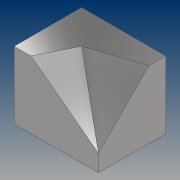
# Autodesk Inventor part: 24
Saved by Autodesk Inventor 2020.2 (Build 242310000, 310)
## iProperties
Created: 2020-09-17
Part Number: 24
Material: 鋼、碳鋼
Document SubType Name: Modeling
Designer: user
Density: 7.85 g/cm^3
Appearance: 半拋光
Mass: 561.275 g
Surface Area: 104.759 cm^2
Volume: 71.5 cm^3
Author: user
Autodesk Inventor part; units mm, degrees
ref_plane "YZ Plane" through (0, 0, 0) normal (1, 0, 0) x (0, 1, 0)
ref_plane "XZ Plane" through (0, 0, 0) normal (0, 1, 0) x (-1, 0, 0)
sketch "草圖1" plane through (0, 0, 0) normal (0, 1, 0) x (-1, 0, 0)
  line L0 (0, 0) -> (-50, 0)
  line L1 (-50, 0) -> (-50, -40)
  line L2 (-50, -40) -> (0, -40)
  line L3 (0, -40) -> (0, 0)
  dimension "d0" = 50
  dimension "d1" = 40
  constraints: 8 end point, 2 parallel, 1 horizontal, 1 perpendicular
  measures "d0" distance of L0.start L0.end
  measures "d1" distance of L2.end L0.start
extrude "擠出1" add sketch "草圖1" along normal blind 40
sketch "草圖2" plane through (0, 40, 0) normal (0, 1, 0) x (1, 0, 0)
  line L0 (0, 0) -> (0, 40) construction
  line L1 (0, 40) -> (50, 40) construction
  line L2 (50, 40) -> (50, 0) construction
  line L3 (50, 0) -> (0, 0) construction
  line L4 (0, 0) -> (50, 0) construction
  line L5 (10, 0) -> (20, 20)
  line L6 (20, 20) -> (50, 0)
  line L7 (10, 0) -> (50, 0)
  dimension "d4" = 20
  dimension "d5" = 40
  dimension "d6" = 10
  constraints: 6 end point, 1 collinear, 1 point on line
  measures "d4" distance from line of L5.end L3
  measures "d5" distance from line of L2 L5.start
  measures "d6" horizontal distance of L5.end L5.start
ref_plane "工作平面1" through (0, 10, 0) normal (0, -1, 0) x (1, 0, 0)
sketch "草圖3" plane through (0, 10, 0) normal (0, -1, 0) x (1, 0, 0)
  line L0 (0, -40) -> (0, 0) construction
  line L1 (0, 0) -> (50, 0) construction
  line L2 (50, 0) -> (50, -40) construction
  line L3 (50, -40) -> (0, -40) construction
  line L4 (0, 0) -> (50, 0) projected
  constraints: 1 coincident
loft "斷面混成1" cut profiles "草圖2" section 2 point at (50, 10, 0)
sketch "草圖4" plane through (0, 40, 0) normal (0, 1, 0) x (1, 0, 0)
  line L0 (50, 0) -> (20, 20) construction
  line L1 (20, 20) -> (10, 0) construction
  line L2 (10, 0) -> (0, 0) construction
  line L3 (0, 0) -> (0, 40) construction
  line L4 (0, 40) -> (50, 40) construction
  line L5 (50, 40) -> (50, 0) construction
  line L6 (20, 20) -> (50, 0) projected
  line L7 (20, 20) -> (50, 30)
  line L8 (50, 0) -> (50, 40) construction
  line L9 (50, 30) -> (50, 0)
  line L10 (10, 0) -> (20, 20) construction
  line L11 (50, 0) -> (20, 20)
  dimension "d12" = 10
  constraints: 6 end point, 1 collinear, 1 point on line
  measures "d12" distance from line of L4 L7.end
sketch "草圖5" plane through (0, 10, 0) normal (0, -1, 0) x (1, 0, 0)
  line L0 (50, 0) -> (50, -40) construction
  point P0 (0, 0)
loft "斷面混成2" cut profiles "草圖4" section 2 point at (50, 10, 0)
